Autodesk Fusion 360 part; units mm, degrees
note: some values were not read from the file. Chosen so that the rebuilt part matches the saved one: which bodies a step acts on; which sketch regions a step uses.
(part 4 of 6)
  line L1579 (-25.4944, -143.9497) -> (-22.9944, -143.9497)
  line L1580 (-92.5268, -139.0331) -> (-91.2768, -141.1981)
  line L1581 (-97.649, -139.0331) -> (-98.899, -136.868)
  line L1582 (-60.9101, -141.1981) -> (-58.4101, -141.1981)
  line L1583 (-1.5, -141.7847) -> (-2.75, -139.6196)
  line L1584 (-53.3611, -133.9529) -> (-55.8611, -133.9529)
  line L1585 (-65.9833, -133.9529) -> (-67.2333, -136.118)
  line L1586 (-36.8667, -141.7847) -> (-35.6167, -143.9497)
  line L1587 (-72.2824, -139.0331) -> (-71.0324, -141.1981)
  line L1588 (-35.6167, -133.9529) -> (-36.8667, -136.118)
  line L1589 (-35.6167, -143.9497) -> (-33.1167, -143.9497)
  line L1590 (-87.4778, -136.118) -> (-86.2278, -138.2831)
  line L1591 (-50.7879, -141.1981) -> (-48.2879, -141.1981)
  line L1592 (-68.5324, -136.868) -> (-71.0324, -136.868)
  line L1593 (-17.9213, -146.8648) -> (-16.6713, -144.6997)
  line L1594 (-86.2278, -133.9529) -> (-87.4778, -136.118)
  line L1595 (-22.9944, -143.9497) -> (-21.7444, -141.7847)
  line L1596 (-31.8667, -141.7847) -> (-33.1167, -139.6196)
  line L1597 (-92.6, -136.118) -> (-93.85, -133.9529)
  line L1598 (-33.1167, -139.6196) -> (-35.6167, -139.6196)
  line L1599 (-2.75, -143.9497) -> (-1.5, -141.7847)
  line L1600 (-2.75, -139.6196) -> (-5.25, -139.6196)
  line L1601 (-33.1167, -143.9497) -> (-31.8667, -141.7847)
  line L1602 (-76.1056, -138.2831) -> (-73.6056, -138.2831)
  line L1603 (-28.0435, -146.8648) -> (-26.7935, -144.6997)
  line L1604 (-63.4833, -133.9529) -> (-65.9833, -133.9529)
  line L1605 (-7.799, -142.5347) -> (-10.299, -142.5347)
  line L1606 (-48.2879, -136.868) -> (-50.7879, -136.868)
  line L1607 (-78.6546, -141.1981) -> (-77.4046, -139.0331)
  line L1608 (-15.3722, -139.6196) -> (-16.6222, -141.7847)
  line L1609 (-101.399, -136.868) -> (-102.649, -139.0331)
  line L1610 (-102.649, -139.0331) -> (-101.399, -141.1981)
  line L1611 (-83.7278, -138.2831) -> (-82.4778, -136.118)
  line L1612 (-77.4046, -139.0331) -> (-78.6546, -136.868)
  line L1613 (-81.1546, -141.1981) -> (-78.6546, -141.1981)
  line L1614 (-40.6657, -136.868) -> (-41.9157, -139.0331)
  line L1615 (-31.7935, -144.6997) -> (-30.5435, -146.8648)
  line L1616 (-57.1111, -136.118) -> (-55.8611, -138.2831)
  line L1617 (-83.7278, -133.9529) -> (-86.2278, -133.9529)
  line L1618 (-93.85, -133.9529) -> (-96.35, -133.9529)
  line L1619 (-21.6713, -144.6997) -> (-20.4213, -146.8648)
  line L1620 (-67.2333, -136.118) -> (-65.9833, -138.2831)
  line L1621 (-86.2278, -138.2831) -> (-83.7278, -138.2831)
  line L1622 (-98.899, -136.868) -> (-101.399, -136.868)
  line L1623 (-21.7444, -141.7847) -> (-22.9944, -139.6196)
  line L1624 (-26.7935, -139.0331) -> (-28.0435, -136.868)
  line L1625 (-16.6713, -144.6997) -> (-17.9213, -142.5347)
  line L1626 (-87.5268, -139.0331) -> (-88.7768, -136.868)
  line L1627 (-88.7768, -141.1981) -> (-87.5268, -139.0331)
  line L1628 (-48.2879, -146.8648) -> (-47.0379, -144.6997)
  line L1629 (-62.2333, -141.7847) -> (-63.4833, -139.6196)
  line L1630 (-15.3722, -143.9497) -> (-12.8722, -143.9497)
  line L1631 (-83.7278, -143.9497) -> (-82.4778, -141.7847)
  line L1632 (-67.2824, -144.6997) -> (-68.5324, -142.5347)
  line L1633 (-77.4046, -144.6997) -> (-78.6546, -142.5347)
  line L1634 (-83.7278, -139.6196) -> (-86.2278, -139.6196)
  line L1635 (-63.4833, -139.6196) -> (-65.9833, -139.6196)
  line L1636 (-47.0379, -144.6997) -> (-48.2879, -142.5347)
  line L1637 (-38.1657, -146.8648) -> (-36.9157, -144.6997)
  line L1638 (-76.1056, -143.9497) -> (-73.6056, -143.9497)
  line L1639 (-82.4778, -136.118) -> (-83.7278, -133.9529)
  line L1640 (-6.549, -144.6997) -> (-7.799, -142.5347)
  line L1641 (-22.9944, -139.6196) -> (-25.4944, -139.6196)
  line L1642 (-60.9101, -142.5347) -> (-62.1601, -144.6997)
  line L1643 (-17.9213, -142.5347) -> (-20.4213, -142.5347)
  line L1644 (-52.1111, -141.7847) -> (-53.3611, -139.6196)
  line L1645 (-5.25, -143.9497) -> (-2.75, -143.9497)
  line L1646 (-96.35, -133.9529) -> (-97.6, -136.118)
  line L1647 (-72.2824, -144.6997) -> (-71.0324, -146.8648)
  line L1648 (-26.7444, -141.7847) -> (-25.4944, -143.9497)
  line L1649 (-88.7768, -136.868) -> (-91.2768, -136.868)
  line L1650 (-46.9889, -141.7847) -> (-45.7389, -143.9497)
  line L1651 (-76.1056, -139.6196) -> (-77.3556, -141.7847)
  line L1652 (-7.799, -146.8648) -> (-6.549, -144.6997)
  line L1653 (-71.0324, -146.8648) -> (-68.5324, -146.8648)
  line L1654 (-77.3556, -141.7847) -> (-76.1056, -143.9497)
  line L1655 (-96.35, -138.2831) -> (-93.85, -138.2831)
  line L1656 (-58.4101, -142.5347) -> (-60.9101, -142.5347)
  line L1657 (-78.6546, -146.8648) -> (-77.4046, -144.6997)
  line L1658 (-86.2278, -139.6196) -> (-87.4778, -141.7847)
  line L1659 (-68.5324, -142.5347) -> (-71.0324, -142.5347)
  line L1660 (-88.7768, -142.5347) -> (-91.2768, -142.5347)
  line L1661 (-5.25, -139.6196) -> (-6.5, -141.7847)
  line L1662 (-101.399, -141.1981) -> (-98.899, -141.1981)
  line L1663 (-91.2768, -142.5347) -> (-92.5268, -144.6997)
  line L1664 (-81.1546, -142.5347) -> (-82.4046, -144.6997)
  line L1665 (-92.5268, -144.6997) -> (-91.2768, -146.8648)
  line L1666 (-16.6222, -141.7847) -> (-15.3722, -143.9497)
  line L1667 (-91.2768, -141.1981) -> (-88.7768, -141.1981)
  line L1668 (-50.7879, -146.8648) -> (-48.2879, -146.8648)
  line L1669 (-73.6056, -139.6196) -> (-76.1056, -139.6196)
  line L1670 (-78.6546, -142.5347) -> (-81.1546, -142.5347)
  line L1671 (-38.1657, -142.5347) -> (-40.6657, -142.5347)
  line L1672 (-73.6056, -143.9497) -> (-72.3556, -141.7847)
  line L1673 (-98.899, -141.1981) -> (-97.649, -139.0331)
  line L1674 (-10.299, -146.8648) -> (-7.799, -146.8648)
  line L1675 (-53.3611, -143.9497) -> (-52.1111, -141.7847)
  line L1676 (-11.6222, -141.7847) -> (-12.8722, -139.6196)
  line L1677 (-68.5324, -146.8648) -> (-67.2824, -144.6997)
  line L1678 (-50.7879, -142.5347) -> (-52.0379, -144.6997)
  line L1679 (-71.0324, -142.5347) -> (-72.2824, -144.6997)
  line L1680 (-67.2333, -141.7847) -> (-65.9833, -143.9497)
  line L1681 (-97.6, -136.118) -> (-96.35, -138.2831)
  line L1682 (-91.2768, -146.8648) -> (-88.7768, -146.8648)
  line L1683 (-53.3611, -139.6196) -> (-55.8611, -139.6196)
  line L1684 (-20.4213, -146.8648) -> (-17.9213, -146.8648)
  line L1685 (-12.8722, -139.6196) -> (-15.3722, -139.6196)
  line L1686 (-36.9157, -144.6997) -> (-38.1657, -142.5347)
  line L1687 (-40.6657, -146.8648) -> (-38.1657, -146.8648)
  line L1688 (-93.85, -138.2831) -> (-92.6, -136.118)
  line L1689 (-72.3556, -141.7847) -> (-73.6056, -139.6196)
  line L1690 (-41.9157, -144.6997) -> (-40.6657, -146.8648)
  line L1691 (-11.549, -144.6997) -> (-10.299, -146.8648)
  line L1692 (-82.4778, -141.7847) -> (-83.7278, -139.6196)
  line L1693 (-36.9157, -150.3664) -> (-38.1657, -148.2013)
  line L1694 (-40.6657, -142.5347) -> (-41.9157, -144.6997)
  line L1695 (-11.6222, -147.4513) -> (-12.8722, -145.2863)
  line L1696 (-5.25, -149.6164) -> (-2.75, -149.6164)
  line L1697 (-82.4046, -144.6997) -> (-81.1546, -146.8648)
  line L1698 (-30.5435, -148.2013) -> (-31.7935, -150.3664)
  line L1699 (-21.7444, -147.4513) -> (-22.9944, -145.2863)
  line L1700 (-98.899, -146.8648) -> (-97.649, -144.6997)
  line L1701 (-20.4213, -148.2013) -> (-21.6713, -150.3664)
  line L1702 (-55.8611, -139.6196) -> (-57.1111, -141.7847)
  line L1703 (-55.8611, -143.9497) -> (-53.3611, -143.9497)
  line L1704 (-45.7389, -139.6196) -> (-46.9889, -141.7847)
  line L1705 (-12.8722, -145.2863) -> (-15.3722, -145.2863)
  line L1706 (-7.799, -148.2013) -> (-10.299, -148.2013)
  line L1707 (-57.1601, -144.6997) -> (-58.4101, -142.5347)
  line L1708 (-1.5, -147.4513) -> (-2.75, -145.2863)
  line L1709 (-81.1546, -146.8648) -> (-78.6546, -146.8648)
  line L1710 (-16.6222, -147.4513) -> (-15.3722, -149.6164)
  line L1711 (-16.6713, -150.3664) -> (-17.9213, -148.2013)
  line L1712 (-12.8722, -149.6164) -> (-11.6222, -147.4513)
  line L1713 (-17.9213, -152.5315) -> (-16.6713, -150.3664)
  line L1714 (-86.2278, -143.9497) -> (-83.7278, -143.9497)
  line L1715 (-33.1167, -149.6164) -> (-31.8667, -147.4513)
  line L1716 (-87.4778, -141.7847) -> (-86.2278, -143.9497)
  line L1717 (-45.7389, -143.9497) -> (-43.2389, -143.9497)
  line L1718 (-93.85, -139.6196) -> (-96.35, -139.6196)
  line L1719 (-63.4833, -143.9497) -> (-62.2333, -141.7847)
  line L1720 (-41.9889, -141.7847) -> (-43.2389, -139.6196)
  line L1721 (-98.899, -142.5347) -> (-101.399, -142.5347)
  line L1722 (-65.9833, -139.6196) -> (-67.2333, -141.7847)
  line L1723 (-92.6, -141.7847) -> (-93.85, -139.6196)
  line L1724 (-46.9889, -147.4513) -> (-45.7389, -149.6164)
  line L1725 (-58.4101, -146.8648) -> (-57.1601, -144.6997)
  line L1726 (-52.0379, -144.6997) -> (-50.7879, -146.8648)
  line L1727 (-38.1657, -152.5315) -> (-36.9157, -150.3664)
  line L1728 (-45.7389, -149.6164) -> (-43.2389, -149.6164)
  line L1729 (-65.9833, -143.9497) -> (-63.4833, -143.9497)
  line L1730 (-40.6657, -148.2013) -> (-41.9157, -150.3664)
  line L1731 (-43.2389, -143.9497) -> (-41.9889, -141.7847)
  line L1732 (-2.75, -145.2863) -> (-5.25, -145.2863)
  line L1733 (-57.1111, -141.7847) -> (-55.8611, -143.9497)
  line L1734 (-22.9944, -145.2863) -> (-25.4944, -145.2863)
  line L1735 (-28.0435, -148.2013) -> (-30.5435, -148.2013)
  line L1736 (-26.7935, -150.3664) -> (-28.0435, -148.2013)
  line L1737 (-38.1657, -148.2013) -> (-40.6657, -148.2013)
  line L1738 (-28.0435, -152.5315) -> (-26.7935, -150.3664)
  line L1739 (-31.8667, -147.4513) -> (-33.1167, -145.2863)
  line L1740 (-15.3722, -149.6164) -> (-12.8722, -149.6164)
  line L1741 (-31.7935, -150.3664) -> (-30.5435, -152.5315)
  line L1742 (-60.9101, -146.8648) -> (-58.4101, -146.8648)
  line L1743 (-101.399, -142.5347) -> (-102.649, -144.6997)
  line L1744 (-97.6, -141.7847) -> (-96.35, -143.9497)
  line L1745 (-48.2879, -142.5347) -> (-50.7879, -142.5347)
  line L1746 (-10.299, -148.2013) -> (-11.549, -150.3664)
  line L1747 (-21.6713, -150.3664) -> (-20.4213, -152.5315)
  line L1748 (-96.35, -143.9497) -> (-93.85, -143.9497)
  line L1749 (-40.6657, -152.5315) -> (-38.1657, -152.5315)
  line L1750 (-6.549, -150.3664) -> (-7.799, -148.2013)
  line L1751 (-62.1601, -144.6997) -> (-60.9101, -146.8648)
  line L1752 (-20.4213, -152.5315) -> (-17.9213, -152.5315)
  line L1753 (-33.1167, -145.2863) -> (-35.6167, -145.2863)
  line L1754 (-6.5, -147.4513) -> (-5.25, -149.6164)
  line L1755 (-43.2389, -139.6196) -> (-45.7389, -139.6196)
  line L1756 (-96.35, -139.6196) -> (-97.6, -141.7847)
  line L1757 (-93.85, -143.9497) -> (-92.6, -141.7847)
  line L1758 (-73.6056, -145.2863) -> (-76.1056, -145.2863)
  line L1759 (-91.2768, -148.2013) -> (-92.5268, -150.3664)
  line L1760 (-48.2879, -148.2013) -> (-50.7879, -148.2013)
  line L1761 (-86.2278, -149.6164) -> (-83.7278, -149.6164)
  line L1762 (-91.2768, -152.5315) -> (-88.7768, -152.5315)
  line L1763 (-52.1111, -147.4513) -> (-53.3611, -145.2863)
  line L1764 (-77.3556, -147.4513) -> (-76.1056, -149.6164)
  line L1765 (-60.9101, -152.5315) -> (-58.4101, -152.5315)
  line L1766 (-72.3556, -147.4513) -> (-73.6056, -145.2863)
  line L1767 (-5.25, -145.2863) -> (-6.5, -147.4513)
  line L1768 (-41.9889, -147.4513) -> (-43.2389, -145.2863)
  line L1769 (-10.299, -152.5315) -> (-7.799, -152.5315)
  line L1770 (-67.2824, -150.3664) -> (-68.5324, -148.2013)
  line L1771 (-35.6167, -149.6164) -> (-33.1167, -149.6164)
  line L1772 (-48.2879, -152.5315) -> (-47.0379, -150.3664)
  line L1773 (-71.0324, -148.2013) -> (-72.2824, -150.3664)
  line L1774 (-43.2389, -145.2863) -> (-45.7389, -145.2863)
  line L1775 (-97.6, -147.4513) -> (-96.35, -149.6164)
  line L1776 (-35.6167, -145.2863) -> (-36.8667, -147.4513)
  line L1777 (-26.7444, -147.4513) -> (-25.4944, -149.6164)
  line L1778 (-87.5268, -144.6997) -> (-88.7768, -142.5347)
  line L1779 (-68.5324, -148.2013) -> (-71.0324, -148.2013)
  line L1780 (-96.35, -149.6164) -> (-93.85, -149.6164)
  line L1781 (-88.7768, -146.8648) -> (-87.5268, -144.6997)
  line L1782 (-93.85, -145.2863) -> (-96.35, -145.2863)
  line L1783 (-62.2333, -147.4513) -> (-63.4833, -145.2863)
  line L1784 (-25.4944, -149.6164) -> (-22.9944, -149.6164)
  line L1785 (-96.35, -145.2863) -> (-97.6, -147.4513)
  line L1786 (-25.4944, -145.2863) -> (-26.7444, -147.4513)
  line L1787 (-92.5268, -150.3664) -> (-91.2768, -152.5315)
  line L1788 (-65.9833, -145.2863) -> (-67.2333, -147.4513)
  line L1789 (-88.7768, -152.5315) -> (-87.5268, -150.3664)
  line L1790 (-50.7879, -148.2013) -> (-52.0379, -150.3664)
  line L1791 (-57.1601, -150.3664) -> (-58.4101, -148.2013)
  line L1792 (-22.9944, -149.6164) -> (-21.7444, -147.4513)
  line L1793 (-58.4101, -148.2013) -> (-60.9101, -148.2013)
  line L1794 (-47.0379, -150.3664) -> (-48.2879, -148.2013)
  line L1795 (-86.2278, -145.2863) -> (-87.4778, -147.4513)
  line L1796 (-87.5268, -150.3664) -> (-88.7768, -148.2013)
  line L1797 (-50.7879, -152.5315) -> (-48.2879, -152.5315)
  line L1798 (-78.6546, -152.5315) -> (-77.4046, -150.3664)
  line L1799 (-93.85, -149.6164) -> (-92.6, -147.4513)
  line L1800 (-82.4778, -147.4513) -> (-83.7278, -145.2863)
  line L1801 (-81.1546, -148.2013) -> (-82.4046, -150.3664)
  line L1802 (-55.8611, -149.6164) -> (-53.3611, -149.6164)
  line L1803 (-7.799, -152.5315) -> (-6.549, -150.3664)
  line L1804 (-101.399, -146.8648) -> (-98.899, -146.8648)
  line L1805 (-17.9213, -148.2013) -> (-20.4213, -148.2013)
  line L1806 (-36.8667, -147.4513) -> (-35.6167, -149.6164)
  line L1807 (-11.549, -150.3664) -> (-10.299, -152.5315)
  line L1808 (-83.7278, -149.6164) -> (-82.4778, -147.4513)
  line L1809 (-58.4101, -152.5315) -> (-57.1601, -150.3664)
  line L1810 (-77.4046, -150.3664) -> (-78.6546, -148.2013)
  line L1811 (-73.6056, -149.6164) -> (-72.3556, -147.4513)
  line L1812 (-41.9157, -150.3664) -> (-40.6657, -152.5315)
  line L1813 (-92.6, -147.4513) -> (-93.85, -145.2863)
  line L1814 (-30.5435, -152.5315) -> (-28.0435, -152.5315)
  line L1815 (-15.3722, -145.2863) -> (-16.6222, -147.4513)
  line L1816 (-57.1111, -147.4513) -> (-55.8611, -149.6164)
  line L1817 (-97.649, -144.6997) -> (-98.899, -142.5347)
  line L1818 (-2.75, -149.6164) -> (-1.5, -147.4513)
  line L1819 (-102.649, -144.6997) -> (-101.399, -146.8648)
  line L1820 (-43.2389, -150.9529) -> (-45.7389, -150.9529)
  line L1821 (-53.3611, -145.2863) -> (-55.8611, -145.2863)
  line L1822 (-11.6222, -153.118) -> (-12.8722, -150.9529)
  line L1823 (-16.6713, -156.0331) -> (-17.9213, -153.868)
  line L1824 (-72.2824, -150.3664) -> (-71.0324, -152.5315)
  line L1825 (-45.7389, -155.2831) -> (-43.2389, -155.2831)
  line L1826 (-25.4944, -150.9529) -> (-26.7444, -153.118)
  line L1827 (-40.6657, -158.1981) -> (-38.1657, -158.1981)
  line L1828 (-45.7389, -150.9529) -> (-46.9889, -153.118)
  line L1829 (-10.299, -153.868) -> (-11.549, -156.0331)
  line L1830 (-81.1546, -152.5315) -> (-78.6546, -152.5315)
  line L1831 (-16.6222, -153.118) -> (-15.3722, -155.2831)
  line L1832 (-48.2879, -153.868) -> (-50.7879, -153.868)
  line L1833 (-71.0324, -152.5315) -> (-68.5324, -152.5315)
  line L1834 (-76.1056, -145.2863) -> (-77.3556, -147.4513)
  line L1835 (-5.25, -150.9529) -> (-6.5, -153.118)
  line L1836 (-43.2389, -149.6164) -> (-41.9889, -147.4513)
  line L1837 (-50.7879, -153.868) -> (-52.0379, -156.0331)
  line L1838 (-52.0379, -156.0331) -> (-50.7879, -158.1981)
  line L1839 (-50.7879, -158.1981) -> (-48.2879, -158.1981)
  line L1840 (-88.7768, -148.2013) -> (-91.2768, -148.2013)
  line L1841 (-30.5435, -158.1981) -> (-28.0435, -158.1981)
  line L1842 (-68.5324, -152.5315) -> (-67.2824, -150.3664)
  line L1843 (-83.7278, -145.2863) -> (-86.2278, -145.2863)
  line L1844 (-53.3611, -149.6164) -> (-52.1111, -147.4513)
  line L1845 (-33.1167, -150.9529) -> (-35.6167, -150.9529)
  line L1846 (-41.9157, -156.0331) -> (-40.6657, -158.1981)
  line L1847 (-46.9889, -153.118) -> (-45.7389, -155.2831)
  line L1848 (-25.4944, -155.2831) -> (-22.9944, -155.2831)
  line L1849 (-102.649, -150.3664) -> (-101.399, -152.5315)
  line L1850 (-35.6167, -150.9529) -> (-36.8667, -153.118)
  line L1851 (-6.5, -153.118) -> (-5.25, -155.2831)
  line L1852 (-7.799, -153.868) -> (-10.299, -153.868)
  line L1853 (-52.0379, -150.3664) -> (-50.7879, -152.5315)
  line L1854 (-26.7444, -153.118) -> (-25.4944, -155.2831)
  line L1855 (-76.1056, -149.6164) -> (-73.6056, -149.6164)
  line L1856 (-87.4778, -147.4513) -> (-86.2278, -149.6164)
  line L1857 (-82.4046, -150.3664) -> (-81.1546, -152.5315)
  line L1858 (-62.1601, -150.3664) -> (-60.9101, -152.5315)
  line L1859 (-35.6167, -155.2831) -> (-33.1167, -155.2831)
  line L1860 (-2.75, -150.9529) -> (-5.25, -150.9529)
  line L1861 (-43.2389, -155.2831) -> (-41.9889, -153.118)
  line L1862 (-31.7935, -156.0331) -> (-30.5435, -158.1981)
  line L1863 (-67.2333, -147.4513) -> (-65.9833, -149.6164)
  line L1864 (-63.4833, -145.2863) -> (-65.9833, -145.2863)
  line L1865 (-36.9157, -156.0331) -> (-38.1657, -153.868)
  line L1866 (-78.6546, -148.2013) -> (-81.1546, -148.2013)
  line L1867 (-28.0435, -153.868) -> (-30.5435, -153.868)
  line L1868 (-41.9889, -153.118) -> (-43.2389, -150.9529)
  line L1869 (-12.8722, -150.9529) -> (-15.3722, -150.9529)
  line L1870 (-15.3722, -150.9529) -> (-16.6222, -153.118)
  line L1871 (-60.9101, -148.2013) -> (-62.1601, -150.3664)
  line L1872 (-38.1657, -158.1981) -> (-36.9157, -156.0331)
  line L1873 (-28.0435, -158.1981) -> (-26.7935, -156.0331)
  line L1874 (-5.25, -155.2831) -> (-2.75, -155.2831)
  line L1875 (-63.4833, -149.6164) -> (-62.2333, -147.4513)
  line L1876 (-45.7389, -145.2863) -> (-46.9889, -147.4513)
  line L1877 (-40.6657, -153.868) -> (-41.9157, -156.0331)
  line L1878 (-1.5, -153.118) -> (-2.75, -150.9529)
  line L1879 (-65.9833, -149.6164) -> (-63.4833, -149.6164)
  line L1880 (-101.399, -152.5315) -> (-98.899, -152.5315)
  line L1881 (-55.8611, -145.2863) -> (-57.1111, -147.4513)
  line L1882 (-20.4213, -158.1981) -> (-17.9213, -158.1981)
  line L1883 (-10.299, -158.1981) -> (-7.799, -158.1981)
  line L1884 (-52.1111, -153.118) -> (-53.3611, -150.9529)
  line L1885 (-21.6713, -156.0331) -> (-20.4213, -158.1981)
  line L1886 (-63.4833, -150.9529) -> (-65.9833, -150.9529)
  line L1887 (-33.1167, -155.2831) -> (-31.8667, -153.118)
  line L1888 (-53.3611, -150.9529) -> (-55.8611, -150.9529)
  line L1889 (-98.899, -152.5315) -> (-97.649, -150.3664)
  line L1890 (-38.1657, -153.868) -> (-40.6657, -153.868)
  line L1891 (-2.75, -155.2831) -> (-1.5, -153.118)
  line L1892 (-6.549, -156.0331) -> (-7.799, -153.868)
  line L1893 (-93.85, -150.9529) -> (-96.35, -150.9529)
  line L1894 (-98.899, -153.868) -> (-101.399, -153.868)
  line L1895 (-31.8667, -153.118) -> (-33.1167, -150.9529)
  line L1896 (-92.6, -153.118) -> (-93.85, -150.9529)
  line L1897 (-101.399, -148.2013) -> (-102.649, -150.3664)
  line L1898 (-101.399, -153.868) -> (-102.649, -156.0331)
  line L1899 (-20.4213, -153.868) -> (-21.6713, -156.0331)
  line L1900 (-22.9944, -150.9529) -> (-25.4944, -150.9529)
  line L1901 (-102.649, -156.0331) -> (-101.399, -158.1981)
  line L1902 (-86.2278, -155.2831) -> (-83.7278, -155.2831)
  line L1903 (-55.8611, -150.9529) -> (-57.1111, -153.118)
  line L1904 (-101.399, -158.1981) -> (-98.899, -158.1981)
  line L1905 (-65.9833, -155.2831) -> (-63.4833, -155.2831)
  line L1906 (-67.2824, -156.0331) -> (-68.5324, -153.868)
  line L1907 (-57.1601, -156.0331) -> (-58.4101, -153.868)
  line L1908 (-73.6056, -155.2831) -> (-72.3556, -153.118)
  line L1909 (-93.85, -155.2831) -> (-92.6, -153.118)
  line L1910 (-76.1056, -155.2831) -> (-73.6056, -155.2831)
  line L1911 (-7.799, -158.1981) -> (-6.549, -156.0331)
  line L1912 (-92.5268, -156.0331) -> (-91.2768, -158.1981)
  line L1913 (-88.7768, -158.1981) -> (-87.5268, -156.0331)
  line L1914 (-83.7278, -150.9529) -> (-86.2278, -150.9529)
  line L1915 (-96.35, -155.2831) -> (-93.85, -155.2831)
  line L1916 (-88.7768, -153.868) -> (-91.2768, -153.868)
  line L1917 (-11.549, -156.0331) -> (-10.299, -158.1981)
  line L1918 (-30.5435, -153.868) -> (-31.7935, -156.0331)
  line L1919 (-98.899, -158.1981) -> (-97.649, -156.0331)
  line L1920 (-6.5, -158.7847) -> (-5.25, -160.9497)
  line L1921 (-72.2824, -156.0331) -> (-71.0324, -158.1981)
  line L1922 (-62.1601, -156.0331) -> (-60.9101, -158.1981)
  line L1923 (-97.649, -150.3664) -> (-98.899, -148.2013)
  line L1924 (-12.8722, -155.2831) -> (-11.6222, -153.118)
  line L1925 (-81.1546, -153.868) -> (-82.4046, -156.0331)
  line L1926 (-98.899, -148.2013) -> (-101.399, -148.2013)
  line L1927 (-22.9944, -155.2831) -> (-21.7444, -153.118)
  line L1928 (-91.2768, -153.868) -> (-92.5268, -156.0331)
  line L1929 (-68.5324, -158.1981) -> (-67.2824, -156.0331)
  line L1930 (-86.2278, -150.9529) -> (-87.4778, -153.118)
  line L1931 (-21.7444, -153.118) -> (-22.9944, -150.9529)
  line L1932 (-17.9213, -158.1981) -> (-16.6713, -156.0331)
  line L1933 (-26.7935, -156.0331) -> (-28.0435, -153.868)
  line L1934 (-87.4778, -153.118) -> (-86.2278, -155.2831)
  line L1935 (-60.9101, -153.868) -> (-62.1601, -156.0331)
  line L1936 (-87.5268, -156.0331) -> (-88.7768, -153.868)
  line L1937 (-36.8667, -153.118) -> (-35.6167, -155.2831)
  line L1938 (-83.7278, -155.2831) -> (-82.4778, -153.118)
  line L1939 (-73.6056, -150.9529) -> (-76.1056, -150.9529)
  line L1940 (-58.4101, -153.868) -> (-60.9101, -153.868)
  line L1941 (-81.1546, -158.1981) -> (-78.6546, -158.1981)
  line L1942 (-17.9213, -153.868) -> (-20.4213, -153.868)
  line L1943 (-91.2768, -158.1981) -> (-88.7768, -158.1981)
  line L1944 (-96.35, -150.9529) -> (-97.6, -153.118)
  line L1945 (-15.3722, -155.2831) -> (-12.8722, -155.2831)
  line L1946 (-63.4833, -155.2831) -> (-62.2333, -153.118)
  line L1947 (-67.2333, -153.118) -> (-65.9833, -155.2831)
  line L1948 (-35.6167, -156.6196) -> (-36.8667, -158.7847)
  line L1949 (-82.4778, -153.118) -> (-83.7278, -150.9529)
  line L1950 (-40.6657, -163.8648) -> (-38.1657, -163.8648)
  line L1951 (-97.6, -153.118) -> (-96.35, -155.2831)
  line L1952 (-36.8667, -158.7847) -> (-35.6167, -160.9497)
  line L1953 (-53.3611, -155.2831) -> (-52.1111, -153.118)
  line L1954 (-71.0324, -153.868) -> (-72.2824, -156.0331)
  line L1955 (-65.9833, -150.9529) -> (-67.2333, -153.118)
  line L1956 (-57.1111, -153.118) -> (-55.8611, -155.2831)
  line L1957 (-5.25, -156.6196) -> (-6.5, -158.7847)
  line L1958 (-21.6713, -161.6997) -> (-20.4213, -163.8648)
  line L1959 (-43.2389, -160.9497) -> (-41.9889, -158.7847)
  line L1960 (-31.8667, -158.7847) -> (-33.1167, -156.6196)
  line L1961 (-72.3556, -153.118) -> (-73.6056, -150.9529)
  line L1962 (-55.8611, -160.9497) -> (-53.3611, -160.9497)
  line L1963 (-38.1657, -159.5347) -> (-40.6657, -159.5347)
  line L1964 (-68.5324, -153.868) -> (-71.0324, -153.868)
  line L1965 (-41.9157, -161.6997) -> (-40.6657, -163.8648)
  line L1966 (-46.9889, -158.7847) -> (-45.7389, -160.9497)
  line L1967 (-22.9944, -160.9497) -> (-21.7444, -158.7847)
  line L1968 (-30.5435, -163.8648) -> (-28.0435, -163.8648)
  line L1969 (-52.1111, -158.7847) -> (-53.3611, -156.6196)
  line L1970 (-7.799, -163.8648) -> (-6.549, -161.6997)
  line L1971 (-20.4213, -163.8648) -> (-17.9213, -163.8648)
  line L1972 (-48.2879, -163.8648) -> (-47.0379, -161.6997)
  line L1973 (-53.3611, -156.6196) -> (-55.8611, -156.6196)
  line L1974 (-55.8611, -156.6196) -> (-57.1111, -158.7847)
  line L1975 (-60.9101, -158.1981) -> (-58.4101, -158.1981)
  line L1976 (-50.7879, -163.8648) -> (-48.2879, -163.8648)
  line L1977 (-10.299, -163.8648) -> (-7.799, -163.8648)
  line L1978 (-78.6546, -153.868) -> (-81.1546, -153.868)
  line L1979 (-10.299, -159.5347) -> (-11.549, -161.6997)
  line L1980 (-12.8722, -156.6196) -> (-15.3722, -156.6196)
  line L1981 (-77.3556, -153.118) -> (-76.1056, -155.2831)
  line L1982 (-82.4046, -156.0331) -> (-81.1546, -158.1981)
  line L1983 (-53.3611, -160.9497) -> (-52.1111, -158.7847)
  line L1984 (-25.4944, -156.6196) -> (-26.7444, -158.7847)
  line L1985 (-7.799, -159.5347) -> (-10.299, -159.5347)
  line L1986 (-43.2389, -156.6196) -> (-45.7389, -156.6196)
  line L1987 (-71.0324, -158.1981) -> (-68.5324, -158.1981)
  line L1988 (-47.0379, -156.0331) -> (-48.2879, -153.868)
  line L1989 (-35.6167, -160.9497) -> (-33.1167, -160.9497)
  line L1990 (-48.2879, -158.1981) -> (-47.0379, -156.0331)
  line L1991 (-55.8611, -155.2831) -> (-53.3611, -155.2831)
  line L1992 (-16.6222, -158.7847) -> (-15.3722, -160.9497)
  line L1993 (-45.7389, -156.6196) -> (-46.9889, -158.7847)
  line L1994 (-31.7935, -161.6997) -> (-30.5435, -163.8648)
  line L1995 (-97.649, -156.0331) -> (-98.899, -153.868)
  line L1996 (-76.1056, -150.9529) -> (-77.3556, -153.118)
  line L1997 (-78.6546, -158.1981) -> (-77.4046, -156.0331)
  line L1998 (-5.25, -160.9497) -> (-2.75, -160.9497)
  line L1999 (-17.9213, -159.5347) -> (-20.4213, -159.5347)
  line L2000 (-16.6713, -161.6997) -> (-17.9213, -159.5347)
  line L2001 (-77.4046, -156.0331) -> (-78.6546, -153.868)
  line L2002 (-57.1111, -158.7847) -> (-55.8611, -160.9497)
  line L2003 (-50.7879, -159.5347) -> (-52.0379, -161.6997)
  line L2004 (-11.549, -161.6997) -> (-10.299, -163.8648)
  line L2005 (-6.549, -161.6997) -> (-7.799, -159.5347)
  line L2006 (-62.2333, -153.118) -> (-63.4833, -150.9529)
  line L2007 (-21.7444, -158.7847) -> (-22.9944, -156.6196)
  line L2008 (-26.7444, -158.7847) -> (-25.4944, -160.9497)
  line L2009 (-58.4101, -158.1981) -> (-57.1601, -156.0331)
  line L2010 (-20.4213, -159.5347) -> (-21.6713, -161.6997)
  line L2011 (-52.0379, -161.6997) -> (-50.7879, -163.8648)
  line L2012 (-77.3556, -158.7847) -> (-76.1056, -160.9497)
  line L2013 (-15.3722, -160.9497) -> (-12.8722, -160.9497)
  line L2014 (-1.5, -164.4513) -> (-2.75, -162.2863)
  line L2015 (-63.4833, -160.9497) -> (-62.2333, -158.7847)
  line L2016 (-11.6222, -158.7847) -> (-12.8722, -156.6196)
  line L2017 (-65.9833, -160.9497) -> (-63.4833, -160.9497)
  line L2018 (-77.4046, -161.6997) -> (-78.6546, -159.5347)
  line L2019 (-93.85, -160.9497) -> (-92.6, -158.7847)
  line L2020 (-96.35, -156.6196) -> (-97.6, -158.7847)
  line L2021 (-81.1546, -163.8648) -> (-78.6546, -163.8648)
  line L2022 (-28.0435, -163.8648) -> (-26.7935, -161.6997)
  line L2023 (-62.2333, -158.7847) -> (-63.4833, -156.6196)
  line L2024 (-88.7768, -163.8648) -> (-87.5268, -161.6997)
  line L2025 (-101.399, -163.8648) -> (-98.899, -163.8648)
  line L2026 (-36.9157, -161.6997) -> (-38.1657, -159.5347)
  line L2027 (-76.1056, -156.6196) -> (-77.3556, -158.7847)
  line L2028 (-97.6, -158.7847) -> (-96.35, -160.9497)
  line L2029 (-57.1601, -161.6997) -> (-58.4101, -159.5347)
  line L2030 (-2.75, -162.2863) -> (-5.25, -162.2863)
  line L2031 (-72.2824, -161.6997) -> (-71.0324, -163.8648)
  line L2032 (-47.0379, -161.6997) -> (-48.2879, -159.5347)
  line L2033 (-86.2278, -160.9497) -> (-83.7278, -160.9497)
  line L2034 (-30.5435, -159.5347) -> (-31.7935, -161.6997)
  line L2035 (-33.1167, -160.9497) -> (-31.8667, -158.7847)
  line L2036 (-48.2879, -159.5347) -> (-50.7879, -159.5347)
  line L2037 (-2.75, -156.6196) -> (-5.25, -156.6196)
  line L2038 (-83.7278, -156.6196) -> (-86.2278, -156.6196)
  line L2039 (-87.5268, -161.6997) -> (-88.7768, -159.5347)
  line L2040 (-92.5268, -161.6997) -> (-91.2768, -163.8648)
  line L2041 (-87.4778, -158.7847) -> (-86.2278, -160.9497)
  line L2042 (-98.899, -163.8648) -> (-97.649, -161.6997)
  line L2043 (-5.25, -166.6164) -> (-2.75, -166.6164)
  line L2044 (-72.3556, -158.7847) -> (-73.6056, -156.6196)
  line L2045 (-1.5, -158.7847) -> (-2.75, -156.6196)
  line L2046 (-96.35, -160.9497) -> (-93.85, -160.9497)
  line L2047 (-26.7935, -161.6997) -> (-28.0435, -159.5347)
  line L2048 (-22.9944, -156.6196) -> (-25.4944, -156.6196)
  line L2049 (-17.9213, -163.8648) -> (-16.6713, -161.6997)
  line L2050 (-38.1657, -163.8648) -> (-36.9157, -161.6997)
  line L2051 (-45.7389, -160.9497) -> (-43.2389, -160.9497)
  line L2052 (-40.6657, -159.5347) -> (-41.9157, -161.6997)
  line L2053 (-91.2768, -163.8648) -> (-88.7768, -163.8648)
  line L2054 (-28.0435, -159.5347) -> (-30.5435, -159.5347)
  line L2055 (-97.649, -161.6997) -> (-98.899, -159.5347)
  line L2056 (-10.299, -165.2013) -> (-11.549, -167.3664)
  line L2057 (-92.6, -158.7847) -> (-93.85, -156.6196)
  line L2058 (-41.9889, -158.7847) -> (-43.2389, -156.6196)
  line L2059 (-91.2768, -159.5347) -> (-92.5268, -161.6997)
  line L2060 (-101.399, -159.5347) -> (-102.649, -161.6997)
  line L2061 (-83.7278, -160.9497) -> (-82.4778, -158.7847)
  line L2062 (-60.9101, -159.5347) -> (-62.1601, -161.6997)
  line L2063 (-71.0324, -159.5347) -> (-72.2824, -161.6997)
  line L2064 (-58.4101, -163.8648) -> (-57.1601, -161.6997)
  line L2065 (-82.4046, -161.6997) -> (-81.1546, -163.8648)
  line L2066 (-6.5, -164.4513) -> (-5.25, -166.6164)
  line L2067 (-15.3722, -156.6196) -> (-16.6222, -158.7847)
  line L2068 (-2.75, -160.9497) -> (-1.5, -158.7847)
  line L2069 (-88.7768, -159.5347) -> (-91.2768, -159.5347)
  line L2070 (-2.75, -166.6164) -> (-1.5, -164.4513)
  line L2071 (-25.4944, -160.9497) -> (-22.9944, -160.9497)
  line L2072 (-33.1167, -156.6196) -> (-35.6167, -156.6196)
  line L2073 (-12.8722, -160.9497) -> (-11.6222, -158.7847)
  line L2074 (-93.85, -156.6196) -> (-96.35, -156.6196)
  line L2075 (-102.649, -161.6997) -> (-101.399, -163.8648)
  line L2076 (-55.8611, -162.2863) -> (-57.1111, -164.4513)
  line L2077 (-50.7879, -165.2013) -> (-52.0379, -167.3664)
  line L2078 (-76.1056, -160.9497) -> (-73.6056, -160.9497)
  line L2079 (-26.7444, -164.4513) -> (-25.4944, -166.6164)
  line L2080 (-16.6713, -167.3664) -> (-17.9213, -165.2013)
  line L2081 (-38.1657, -165.2013) -> (-40.6657, -165.2013)
  line L2082 (-68.5324, -163.8648) -> (-67.2824, -161.6997)
  line L2083 (-17.9213, -169.5315) -> (-16.6713, -167.3664)
  line L2084 (-25.4944, -162.2863) -> (-26.7444, -164.4513)
  line L2085 (-47.0379, -167.3664) -> (-48.2879, -165.2013)
  line L2086 (-58.4101, -159.5347) -> (-60.9101, -159.5347)
  line L2087 (-53.3611, -166.6164) -> (-52.1111, -164.4513)
  line L2088 (-52.1111, -164.4513) -> (-53.3611, -162.2863)
  line L2089 (-60.9101, -163.8648) -> (-58.4101, -163.8648)
  line L2090 (-63.4833, -156.6196) -> (-65.9833, -156.6196)
  line L2091 (-30.5435, -169.5315) -> (-28.0435, -169.5315)
  line L2092 (-58.4101, -165.2013) -> (-60.9101, -165.2013)
  line L2093 (-45.7389, -166.6164) -> (-43.2389, -166.6164)
  line L2094 (-30.5435, -165.2013) -> (-31.7935, -167.3664)
  line L2095 (-60.9101, -169.5315) -> (-58.4101, -169.5315)
  line L2096 (-43.2389, -166.6164) -> (-41.9889, -164.4513)
  line L2097 (-58.4101, -169.5315) -> (-57.1601, -167.3664)
  line L2098 (-81.1546, -159.5347) -> (-82.4046, -161.6997)
  line L2099 (-62.1601, -167.3664) -> (-60.9101, -169.5315)
  line L2100 (-35.6167, -162.2863) -> (-36.8667, -164.4513)
  line L2101 (-86.2278, -156.6196) -> (-87.4778, -158.7847)
  line L2102 (-55.8611, -166.6164) -> (-53.3611, -166.6164)
  line L2103 (-53.3611, -162.2863) -> (-55.8611, -162.2863)
  line L2104 (-45.7389, -162.2863) -> (-46.9889, -164.4513)
  line L2105 (-11.549, -167.3664) -> (-10.299, -169.5315)
  line L2106 (-38.1657, -169.5315) -> (-36.9157, -167.3664)
  line L2107 (-36.8667, -164.4513) -> (-35.6167, -166.6164)
  line L2108 (-15.3722, -162.2863) -> (-16.6222, -164.4513)
  line L2109 (-48.2879, -169.5315) -> (-47.0379, -167.3664)
  line L2110 (-60.9101, -165.2013) -> (-62.1601, -167.3664)
  line L2111 (-21.6713, -167.3664) -> (-20.4213, -169.5315)
  line L2112 (-11.6222, -164.4513) -> (-12.8722, -162.2863)
  line L2113 (-62.1601, -161.6997) -> (-60.9101, -163.8648)
  line L2114 (-73.6056, -156.6196) -> (-76.1056, -156.6196)
  line L2115 (-67.2333, -158.7847) -> (-65.9833, -160.9497)
  line L2116 (-26.7935, -167.3664) -> (-28.0435, -165.2013)
  line L2117 (-48.2879, -165.2013) -> (-50.7879, -165.2013)
  line L2118 (-65.9833, -156.6196) -> (-67.2333, -158.7847)
  line L2119 (-98.899, -159.5347) -> (-101.399, -159.5347)
  line L2120 (-78.6546, -163.8648) -> (-77.4046, -161.6997)
  line L2121 (-22.9944, -162.2863) -> (-25.4944, -162.2863)
  line L2122 (-40.6657, -165.2013) -> (-41.9157, -167.3664)
  line L2123 (-5.25, -162.2863) -> (-6.5, -164.4513)
  line L2124 (-7.799, -165.2013) -> (-10.299, -165.2013)
  line L2125 (-67.2824, -161.6997) -> (-68.5324, -159.5347)
  line L2126 (-33.1167, -162.2863) -> (-35.6167, -162.2863)
  line L2127 (-31.7935, -167.3664) -> (-30.5435, -169.5315)
  line L2128 (-40.6657, -169.5315) -> (-38.1657, -169.5315)
  line L2129 (-12.8722, -166.6164) -> (-11.6222, -164.4513)
  line L2130 (-12.8722, -162.2863) -> (-15.3722, -162.2863)
  line L2131 (-41.9157, -167.3664) -> (-40.6657, -169.5315)
  line L2132 (-46.9889, -164.4513) -> (-45.7389, -166.6164)
  line L2133 (-41.9889, -164.4513) -> (-43.2389, -162.2863)
  line L2134 (-68.5324, -159.5347) -> (-71.0324, -159.5347)
  line L2135 (-73.6056, -160.9497) -> (-72.3556, -158.7847)
  line L2136 (-82.4778, -158.7847) -> (-83.7278, -156.6196)
  line L2137 (-71.0324, -163.8648) -> (-68.5324, -163.8648)
  line L2138 (-78.6546, -159.5347) -> (-81.1546, -159.5347)
  line L2139 (-10.299, -169.5315) -> (-7.799, -169.5315)
  line L2140 (-28.0435, -169.5315) -> (-26.7935, -167.3664)
  line L2141 (-15.3722, -166.6164) -> (-12.8722, -166.6164)
  line L2142 (-73.6056, -162.2863) -> (-76.1056, -162.2863)
  line L2143 (-98.899, -169.5315) -> (-97.649, -167.3664)
  line L2144 (-82.4778, -164.4513) -> (-83.7278, -162.2863)
  line L2145 (-88.7768, -169.5315) -> (-87.5268, -167.3664)
  line L2146 (-86.2278, -162.2863) -> (-87.4778, -164.4513)
  line L2147 (-102.649, -167.3664) -> (-101.399, -169.5315)
  line L2148 (-63.4833, -166.6164) -> (-62.2333, -164.4513)
  line L2149 (-91.2768, -169.5315) -> (-88.7768, -169.5315)
  line L2150 (-81.1546, -169.5315) -> (-78.6546, -169.5315)
  line L2151 (-7.799, -169.5315) -> (-6.549, -167.3664)
  line L2152 (-68.5324, -169.5315) -> (-67.2824, -167.3664)
  line L2153 (-17.9213, -165.2013) -> (-20.4213, -165.2013)
  line L2154 (-91.2768, -165.2013) -> (-92.5268, -167.3664)
  line L2155 (-52.0379, -167.3664) -> (-50.7879, -169.5315)
  line L2156 (-65.9833, -162.2863) -> (-67.2333, -164.4513)
  line L2157 (-83.7278, -166.6164) -> (-82.4778, -164.4513)
  line L2158 (-68.5324, -165.2013) -> (-71.0324, -165.2013)
  line L2159 (-81.1546, -165.2013) -> (-82.4046, -167.3664)
  line L2160 (-57.1601, -167.3664) -> (-58.4101, -165.2013)
  line L2161 (-20.4213, -169.5315) -> (-17.9213, -169.5315)
  line L2162 (-21.7444, -164.4513) -> (-22.9944, -162.2863)
  line L2163 (-86.2278, -166.6164) -> (-83.7278, -166.6164)
  line L2164 (-96.35, -166.6164) -> (-93.85, -166.6164)
  line L2165 (-22.9944, -166.6164) -> (-21.7444, -164.4513)
  line L2166 (-67.2824, -167.3664) -> (-68.5324, -165.2013)
  line L2167 (-93.85, -166.6164) -> (-92.6, -164.4513)
  line L2168 (-20.4213, -165.2013) -> (-21.6713, -167.3664)
  line L2169 (-83.7278, -162.2863) -> (-86.2278, -162.2863)
  line L2170 (-6.549, -167.3664) -> (-7.799, -165.2013)
  line L2171 (-93.85, -162.2863) -> (-96.35, -162.2863)
  line L2172 (-82.4046, -167.3664) -> (-81.1546, -169.5315)
  line L2173 (-101.399, -165.2013) -> (-102.649, -167.3664)
  line L2174 (-101.399, -169.5315) -> (-98.899, -169.5315)
  line L2175 (-98.899, -165.2013) -> (-101.399, -165.2013)
  line L2176 (-50.7879, -169.5315) -> (-48.2879, -169.5315)
  line L2177 (-97.649, -167.3664) -> (-98.899, -165.2013)
  line L2178 (-63.4833, -162.2863) -> (-65.9833, -162.2863)
  line L2179 (-71.0324, -169.5315) -> (-68.5324, -169.5315)
  line L2180 (-96.35, -162.2863) -> (-97.6, -164.4513)
  line L2181 (-72.2824, -167.3664) -> (-71.0324, -169.5315)
  line L2182 (-88.7768, -165.2013) -> (-91.2768, -165.2013)
  line L2183 (-77.3556, -164.4513) -> (-76.1056, -166.6164)
  line L2184 (-97.6, -164.4513) -> (-96.35, -166.6164)
  line L2185 (-92.6, -164.4513) -> (-93.85, -162.2863)
  line L2186 (-76.1056, -162.2863) -> (-77.3556, -164.4513)
  line L2187 (-25.4944, -166.6164) -> (-22.9944, -166.6164)
  line L2188 (-28.0435, -165.2013) -> (-30.5435, -165.2013)
  line L2189 (-31.8667, -164.4513) -> (-33.1167, -162.2863)
  line L2190 (-35.6167, -166.6164) -> (-33.1167, -166.6164)
  line L2191 (-16.6222, -164.4513) -> (-15.3722, -166.6164)
  line L2192 (-78.6546, -165.2013) -> (-81.1546, -165.2013)
  line L2193 (-76.1056, -166.6164) -> (-73.6056, -166.6164)
  line L2194 (-72.3556, -164.4513) -> (-73.6056, -162.2863)
  line L2195 (-92.5268, -167.3664) -> (-91.2768, -169.5315)
  line L2196 (-67.2333, -164.4513) -> (-65.9833, -166.6164)
  line L2197 (-87.5268, -167.3664) -> (-88.7768, -165.2013)
  line L2198 (-57.1111, -164.4513) -> (-55.8611, -166.6164)
  line L2199 (-43.2389, -162.2863) -> (-45.7389, -162.2863)
  line L2200 (-71.0324, -165.2013) -> (-72.2824, -167.3664)
  line L2201 (-65.9833, -166.6164) -> (-63.4833, -166.6164)
  line L2202 (-33.1167, -166.6164) -> (-31.8667, -164.4513)
  line L2203 (-36.9157, -167.3664) -> (-38.1657, -165.2013)
  line L2204 (-87.4778, -164.4513) -> (-86.2278, -166.6164)
  line L2205 (-78.6546, -169.5315) -> (-77.4046, -167.3664)
  line L2206 (-73.6056, -166.6164) -> (-72.3556, -164.4513)
  line L2207 (-77.4046, -167.3664) -> (-78.6546, -165.2013)
  line L2208 (-62.2333, -164.4513) -> (-63.4833, -162.2863)
  line L2209 (-11.549, -76.6997) -> (-10.299, -78.8648)
  line L2210 (-30.5435, -74.5347) -> (-31.7935, -76.6997)
  line L2211 (-41.9889, -73.7847) -> (-43.2389, -71.6196)
  line L2212 (-31.7935, -76.6997) -> (-30.5435, -78.8648)
  line L2213 (-36.9157, -76.6997) -> (-38.1657, -74.5347)
  line L2214 (-87.5268, -71.0331) -> (-88.7768, -68.868)
  line L2215 (-57.1111, -73.7847) -> (-55.8611, -75.9497)
  line L2216 (-10.299, -78.8648) -> (-7.799, -78.8648)
  line L2217 (-2.75, -75.9497) -> (-1.5, -73.7847)
  line L2218 (-26.7935, -76.6997) -> (-28.0435, -74.5347)
  line L2219 (-22.9944, -75.9497) -> (-21.7444, -73.7847)
  line L2220 (-6.5, -73.7847) -> (-5.25, -75.9497)
  line L2221 (-20.4213, -78.8648) -> (-17.9213, -78.8648)
  line L2222 (-17.9213, -78.8648) -> (-16.6713, -76.6997)
  line L2223 (-97.649, -71.0331) -> (-98.899, -68.868)
  line L2224 (-28.0435, -78.8648) -> (-26.7935, -76.6997)
  line L2225 (-38.1657, -74.5347) -> (-40.6657, -74.5347)
  line L2226 (-35.6167, -75.9497) -> (-33.1167, -75.9497)
  line L2227 (-21.7444, -73.7847) -> (-22.9944, -71.6196)
  line L2228 (-98.899, -73.1981) -> (-97.649, -71.0331)
  line L2229 (-25.4944, -71.6196) -> (-26.7444, -73.7847)
  line L2230 (-88.7768, -73.1981) -> (-87.5268, -71.0331)
  line L2231 (-12.8722, -71.6196) -> (-15.3722, -71.6196)
  line L2232 (-17.9213, -74.5347) -> (-20.4213, -74.5347)
  line L2233 (-36.8667, -73.7847) -> (-35.6167, -75.9497)
  line L2234 (-101.399, -73.1981) -> (-98.899, -73.1981)
  line L2235 (-97.6, -68.118) -> (-96.35, -70.2831)
  line L2236 (-40.6657, -74.5347) -> (-41.9157, -76.6997)
  line L2237 (-41.9157, -76.6997) -> (-40.6657, -78.8648)
  line L2238 (-38.1657, -78.8648) -> (-36.9157, -76.6997)
  line L2239 (-35.6167, -71.6196) -> (-36.8667, -73.7847)
  line L2240 (-31.8667, -73.7847) -> (-33.1167, -71.6196)
  line L2241 (-43.2389, -75.9497) -> (-41.9889, -73.7847)
  line L2242 (-2.75, -71.6196) -> (-5.25, -71.6196)
  line L2243 (-16.6222, -73.7847) -> (-15.3722, -75.9497)
  line L2244 (-55.8611, -75.9497) -> (-53.3611, -75.9497)
  line L2245 (-46.9889, -73.7847) -> (-45.7389, -75.9497)
  line L2246 (-48.2879, -78.8648) -> (-47.0379, -76.6997)
  line L2247 (-25.4944, -70.2831) -> (-22.9944, -70.2831)
  line L2248 (-98.899, -68.868) -> (-101.399, -68.868)
  line L2249 (-45.7389, -75.9497) -> (-43.2389, -75.9497)
  line L2250 (-28.0435, -74.5347) -> (-30.5435, -74.5347)
  line L2251 (-20.4213, -74.5347) -> (-21.6713, -76.6997)
  line L2252 (-7.799, -78.8648) -> (-6.549, -76.6997)
  line L2253 (-33.1167, -75.9497) -> (-31.8667, -73.7847)
  line L2254 (-6.549, -76.6997) -> (-7.799, -74.5347)
  line L2255 (-1.5, -73.7847) -> (-2.75, -71.6196)
  line L2256 (-5.25, -71.6196) -> (-6.5, -73.7847)
  line L2257 (-5.25, -75.9497) -> (-2.75, -75.9497)
  line L2258 (-12.8722, -75.9497) -> (-11.6222, -73.7847)
  line L2259 (-25.4944, -75.9497) -> (-22.9944, -75.9497)
  line L2260 (-26.7444, -73.7847) -> (-25.4944, -75.9497)
  line L2261 (-10.299, -74.5347) -> (-11.549, -76.6997)
  line L2262 (-21.6713, -76.6997) -> (-20.4213, -78.8648)
  line L2263 (-16.6713, -76.6997) -> (-17.9213, -74.5347)
  line L2264 (-30.5435, -78.8648) -> (-28.0435, -78.8648)
  line L2265 (-22.9944, -71.6196) -> (-25.4944, -71.6196)
  line L2266 (-33.1167, -71.6196) -> (-35.6167, -71.6196)
  line L2267 (-7.799, -74.5347) -> (-10.299, -74.5347)
  line L2268 (-40.6657, -78.8648) -> (-38.1657, -78.8648)
  line L2269 (-47.0379, -76.6997) -> (-48.2879, -74.5347)
  line L2270 (-15.3722, -71.6196) -> (-16.6222, -73.7847)
  line L2271 (-11.6222, -73.7847) -> (-12.8722, -71.6196)
  line L2272 (-15.3722, -75.9497) -> (-12.8722, -75.9497)
  line L2273 (-101.399, -67.5315) -> (-98.899, -67.5315)
  line L2274 (-43.2389, -70.2831) -> (-41.9889, -68.118)
  line L2275 (-97.649, -65.3664) -> (-98.899, -63.2013)
  line L2276 (-35.6167, -65.9529) -> (-36.8667, -68.118)
  line L2277 (-45.7389, -70.2831) -> (-43.2389, -70.2831)
  line L2278 (-1.5, -68.118) -> (-2.75, -65.9529)
  line L2279 (-97.6, -62.4513) -> (-96.35, -64.6164)
  line L2280 (-40.6657, -68.868) -> (-41.9157, -71.0331)
  line L2281 (-30.5435, -73.1981) -> (-28.0435, -73.1981)
  line L2282 (-15.3722, -65.9529) -> (-16.6222, -68.118)
  line L2283 (-20.4213, -73.1981) -> (-17.9213, -73.1981)
  line L2284 (-33.1167, -65.9529) -> (-35.6167, -65.9529)
  line L2285 (-11.6222, -68.118) -> (-12.8722, -65.9529)
  line L2286 (-5.25, -70.2831) -> (-2.75, -70.2831)
  line L2287 (-28.0435, -73.1981) -> (-26.7935, -71.0331)
  line L2288 (-35.6167, -70.2831) -> (-33.1167, -70.2831)
  line L2289 (-93.85, -60.2863) -> (-96.35, -60.2863)
  line L2290 (-5.25, -65.9529) -> (-6.5, -68.118)
  line L2291 (-17.9213, -73.1981) -> (-16.6713, -71.0331)
  line L2292 (-12.8722, -70.2831) -> (-11.6222, -68.118)
  line L2293 (-30.5435, -68.868) -> (-31.7935, -71.0331)
  line L2294 (-25.4944, -65.9529) -> (-26.7444, -68.118)
  line L2295 (-7.799, -68.868) -> (-10.299, -68.868)
  line L2296 (-31.7935, -71.0331) -> (-30.5435, -73.1981)
  line L2297 (-16.6222, -68.118) -> (-15.3722, -70.2831)
  line L2298 (-22.9944, -70.2831) -> (-21.7444, -68.118)
  line L2299 (-38.1657, -73.1981) -> (-36.9157, -71.0331)
  line L2300 (-2.75, -65.9529) -> (-5.25, -65.9529)
  line L2301 (-36.9157, -71.0331) -> (-38.1657, -68.868)
  line L2302 (-6.549, -71.0331) -> (-7.799, -68.868)
  line L2303 (-12.8722, -65.9529) -> (-15.3722, -65.9529)
  line L2304 (-15.3722, -70.2831) -> (-12.8722, -70.2831)
  line L2305 (-36.8667, -68.118) -> (-35.6167, -70.2831)
  line L2306 (-10.299, -68.868) -> (-11.549, -71.0331)
  line L2307 (-33.1167, -70.2831) -> (-31.8667, -68.118)
  line L2308 (-21.7444, -68.118) -> (-22.9944, -65.9529)
  line L2309 (-16.6713, -71.0331) -> (-17.9213, -68.868)
  line L2310 (-98.899, -63.2013) -> (-101.399, -63.2013)
  line L2311 (-26.7935, -71.0331) -> (-28.0435, -68.868)
  line L2312 (-7.799, -73.1981) -> (-6.549, -71.0331)
  line L2313 (-2.75, -70.2831) -> (-1.5, -68.118)
  line L2314 (-31.8667, -68.118) -> (-33.1167, -65.9529)
  line L2315 (-93.85, -64.6164) -> (-92.6, -62.4513)
  line L2316 (-98.899, -67.5315) -> (-97.649, -65.3664)
  line L2317 (-96.35, -64.6164) -> (-93.85, -64.6164)
  line L2318 (-92.6, -62.4513) -> (-93.85, -60.2863)
  line L2319 (-87.5268, -65.3664) -> (-88.7768, -63.2013)
  line L2320 (-17.9213, -68.868) -> (-20.4213, -68.868)
  line L2321 (-26.7444, -68.118) -> (-25.4944, -70.2831)
  line L2322 (-11.549, -71.0331) -> (-10.299, -73.1981)
  line L2323 (-41.9157, -71.0331) -> (-40.6657, -73.1981)
  line L2324 (-46.9889, -68.118) -> (-45.7389, -70.2831)
  line L2325 (-102.649, -65.3664) -> (-101.399, -67.5315)
  line L2326 (-10.299, -73.1981) -> (-7.799, -73.1981)
  line L2327 (-96.35, -60.2863) -> (-97.6, -62.4513)
  line L2328 (-22.9944, -65.9529) -> (-25.4944, -65.9529)
  line L2329 (-6.5, -68.118) -> (-5.25, -70.2831)
  line L2330 (-101.399, -63.2013) -> (-102.649, -65.3664)
  line L2331 (-28.0435, -68.868) -> (-30.5435, -68.868)
  line L2332 (-38.1657, -68.868) -> (-40.6657, -68.868)
  line L2333 (-21.6713, -71.0331) -> (-20.4213, -73.1981)
  line L2334 (-93.85, -13.6164) -> (-92.6, -11.4513)
  line L2335 (-20.4213, -68.868) -> (-21.6713, -71.0331)
  line L2336 (-40.6657, -73.1981) -> (-38.1657, -73.1981)
  line L2337 (-22.9944, -19.2831) -> (-21.7444, -17.118)
  line L2338 (-1.5, -17.118) -> (-2.75, -14.9529)
  line L2339 (-45.7389, -14.9529) -> (-46.9889, -17.118)
  line L2340 (-41.9889, -17.118) -> (-43.2389, -14.9529)
  line L2341 (-97.649, -14.3664) -> (-98.899, -12.2013)
  line L2342 (-5.25, -14.9529) -> (-6.5, -17.118)
  line L2343 (-93.85, -9.2863) -> (-96.35, -9.2863)
  line L2344 (-22.9944, -14.9529) -> (-25.4944, -14.9529)
  line L2345 (-21.6713, -20.0331) -> (-20.4213, -22.1981)
  line L2346 (-16.6222, -17.118) -> (-15.3722, -19.2831)
  line L2347 (-40.6657, -22.1981) -> (-38.1657, -22.1981)
  line L2348 (-86.2278, -9.2863) -> (-87.4778, -11.4513)
  line L2349 (-92.5268, -14.3664) -> (-91.2768, -16.5315)
  line L2350 (-10.299, -22.1981) -> (-7.799, -22.1981)
  line L2351 (-96.35, -9.2863) -> (-97.6, -11.4513)
  line L2352 (-25.4944, -19.2831) -> (-22.9944, -19.2831)
  line L2353 (-16.6713, -20.0331) -> (-17.9213, -17.868)
  line L2354 (-46.9889, -17.118) -> (-45.7389, -19.2831)
  line L2355 (-101.399, -16.5315) -> (-98.899, -16.5315)
  line L2356 (-48.2879, -17.868) -> (-50.7879, -17.868)
  line L2357 (-36.9157, -20.0331) -> (-38.1657, -17.868)
  line L2358 (-10.299, -17.868) -> (-11.549, -20.0331)
  line L2359 (-50.7879, -17.868) -> (-52.0379, -20.0331)
  line L2360 (-20.4213, -17.868) -> (-21.6713, -20.0331)
  line L2361 (-11.549, -20.0331) -> (-10.299, -22.1981)
  line L2362 (-15.3722, -19.2831) -> (-12.8722, -19.2831)
  line L2363 (-38.1657, -17.868) -> (-40.6657, -17.868)
  line L2364 (-11.6222, -17.118) -> (-12.8722, -14.9529)
  line L2365 (-33.1167, -14.9529) -> (-35.6167, -14.9529)
  line L2366 (-45.7389, -19.2831) -> (-43.2389, -19.2831)
  line L2367 (-87.5268, -14.3664) -> (-88.7768, -12.2013)
  line L2368 (-91.2768, -16.5315) -> (-88.7768, -16.5315)
  line L2369 (-7.799, -22.1981) -> (-6.549, -20.0331)
  line L2370 (-21.7444, -17.118) -> (-22.9944, -14.9529)
  line L2371 (-98.899, -12.2013) -> (-101.399, -12.2013)
  line L2372 (-15.3722, -14.9529) -> (-16.6222, -17.118)
  line L2373 (-31.7935, -20.0331) -> (-30.5435, -22.1981)
  line L2374 (-30.5435, -17.868) -> (-31.7935, -20.0331)
  line L2375 (-35.6167, -14.9529) -> (-36.8667, -17.118)
  line L2376 (-36.8667, -17.118) -> (-35.6167, -19.2831)
  line L2377 (-91.2768, -12.2013) -> (-92.5268, -14.3664)
  line L2378 (-33.1167, -19.2831) -> (-31.8667, -17.118)
  line L2379 (-92.6, -11.4513) -> (-93.85, -9.2863)
  line L2380 (-20.4213, -22.1981) -> (-17.9213, -22.1981)
  line L2381 (-26.7444, -17.118) -> (-25.4944, -19.2831)
  line L2382 (-30.5435, -22.1981) -> (-28.0435, -22.1981)
  line L2383 (-28.0435, -17.868) -> (-30.5435, -17.868)
  line L2384 (-28.0435, -22.1981) -> (-26.7935, -20.0331)
  line L2385 (-43.2389, -14.9529) -> (-45.7389, -14.9529)
  line L2386 (-26.7935, -20.0331) -> (-28.0435, -17.868)
  line L2387 (-43.2389, -19.2831) -> (-41.9889, -17.118)
  line L2388 (-6.549, -20.0331) -> (-7.799, -17.868)
  line L2389 (-17.9213, -17.868) -> (-20.4213, -17.868)
  line L2390 (-25.4944, -14.9529) -> (-26.7444, -17.118)
  line L2391 (-88.7768, -16.5315) -> (-87.5268, -14.3664)
  line L2392 (-35.6167, -19.2831) -> (-33.1167, -19.2831)
  line L2393 (-38.1657, -22.1981) -> (-36.9157, -20.0331)
  line L2394 (-41.9157, -20.0331) -> (-40.6657, -22.1981)
  line L2395 (-17.9213, -22.1981) -> (-16.6713, -20.0331)
  line L2396 (-12.8722, -14.9529) -> (-15.3722, -14.9529)
  line L2397 (-2.75, -14.9529) -> (-5.25, -14.9529)
  line L2398 (-88.7768, -12.2013) -> (-91.2768, -12.2013)
  line L2399 (-97.6, -11.4513) -> (-96.35, -13.6164)
  line L2400 (-96.35, -13.6164) -> (-93.85, -13.6164)
  line L2401 (-91.2768, -22.1981) -> (-88.7768, -22.1981)
  line L2402 (-77.4046, -20.0331) -> (-78.6546, -17.868)
  line L2403 (-98.899, -17.868) -> (-101.399, -17.868)
  line L2404 (-67.2333, -17.118) -> (-65.9833, -19.2831)
  line L2405 (-101.399, -12.2013) -> (-102.649, -14.3664)
  line L2406 (-76.1056, -19.2831) -> (-73.6056, -19.2831)
  line L2407 (-86.2278, -14.9529) -> (-87.4778, -17.118)
  line L2408 (-52.0379, -20.0331) -> (-50.7879, -22.1981)
  line L2409 (-12.8722, -19.2831) -> (-11.6222, -17.118)
  line L2410 (-76.1056, -14.9529) -> (-77.3556, -17.118)
  line L2411 (-2.75, -19.2831) -> (-1.5, -17.118)
  line L2412 (-97.6, -17.118) -> (-96.35, -19.2831)
  line L2413 (-65.9833, -14.9529) -> (-67.2333, -17.118)
  line L2414 (-68.5324, -22.1981) -> (-67.2824, -20.0331)
  line L2415 (-102.649, -14.3664) -> (-101.399, -16.5315)
  line L2416 (-40.6657, -17.868) -> (-41.9157, -20.0331)
  line L2417 (-72.3556, -17.118) -> (-73.6056, -14.9529)
  line L2418 (-52.1111, -17.118) -> (-53.3611, -14.9529)
  line L2419 (-63.4833, -14.9529) -> (-65.9833, -14.9529)
  line L2420 (-60.9101, -22.1981) -> (-58.4101, -22.1981)
  line L2421 (-102.649, -20.0331) -> (-101.399, -22.1981)
  line L2422 (-78.6546, -17.868) -> (-81.1546, -17.868)
  line L2423 (-101.399, -22.1981) -> (-98.899, -22.1981)
  line L2424 (-53.3611, -14.9529) -> (-55.8611, -14.9529)
  line L2425 (-60.9101, -17.868) -> (-62.1601, -20.0331)
  line L2426 (-73.6056, -14.9529) -> (-76.1056, -14.9529)
  line L2427 (-31.8667, -17.118) -> (-33.1167, -14.9529)
  line L2428 (-83.7278, -19.2831) -> (-82.4778, -17.118)
  line L2429 (-83.7278, -14.9529) -> (-86.2278, -14.9529)
  line L2430 (-87.5268, -20.0331) -> (-88.7768, -17.868)